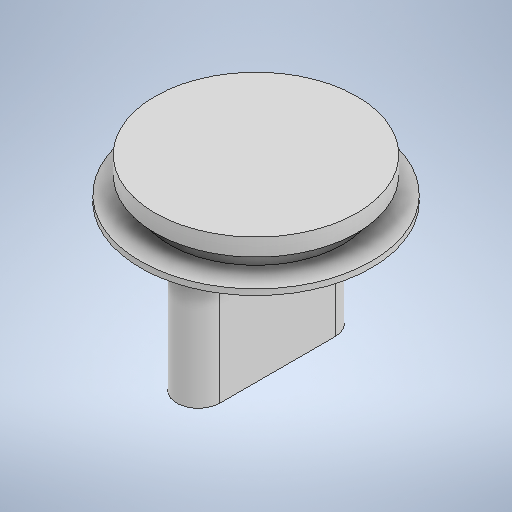
# Autodesk Inventor part: Pin Hole Lock
Saved by Autodesk Inventor 2025 (Build 290162010, 162A)
## iProperties
Created: 2024-06-11
Part Number: Pin Hole Lock
Material: Generic
Document SubType Name: Modeling
Designer: vncnt
Density: 1 g/cm^3
Appearance: Default
Author: vncnt
Autodesk Inventor part; units mm, degrees
ref_plane "YZ Plane" through (0, 0, 0) normal (1, 0, 0) x (0, 1, 0)
ref_plane "XZ Plane" through (0, 0, 0) normal (0, 1, 0) x (-1, 0, 0)
ref_plane "XY Plane" through (0, 0, 0) normal (0, 0, 1) x (1, 0, 0)
sketch "Sketch1" plane through (0, 0, 0) normal (0, 1, 0) x (-1, 0, 0)
  circle A0 centre (0, 0) radius 1.905
  dimension "d0" = 3.81
  constraints: 1 centre point, 1 coincident
  measures "d0" diameter of A0
extrude "Extrusion1" add sketch "Sketch1" along normal blind 2.341
sketch "Sketch2" plane through (0, 2.341, 0) normal (0, 1, 0) x (1, 0, 0)
  circle A0 centre (0, 0) radius 2
  dimension "d3" = 4
  constraints: 1 centre point, 1 coincident
  measures "d3" diameter of A0
extrude "Extrusion2" add sketch "Sketch2" along normal blind 0.1
sketch "Sketch8" plane through (0, 0, 0) normal (0, -1, 0) x (1, 0, 0)
  line L0 (0, 1) -> (0, -1) construction
  line L1 (-0.375, 1) -> (-0.375, -1)
  line L2 (0.375, -1) -> (0.375, 1)
  arc A0 (0.375, 1) -> (-0.375, 1) centre (0, 1) ccw
  arc A1 (-0.375, -1) -> (0.375, -1) centre (0, -1) ccw
  circle A2 centre (0, 0) radius 1.905
  dimension "d22" = 1
  dimension "d23" = 0.75
  constraints: 8 end point, 4 point on circle, 4 tangent, 3 centre point, 1 coincident, 1 midpoint, 1 parallel, 1 vertical
  measures "d22" distance of point (0, 0) L0.end
  measures "d23" diameter of A1
extrude "Extrusion4" cut sketch "Sketch8" against normal up to surface (2.341 mm away)
sketch "Sketch9" plane through (0, 2.441, 0) normal (0, 1, 0) x (1, 0, 0)
  circle A0 centre (0, 0) radius 1.5
  dimension "d26" = 3
  constraints: 1 centre point, 1 coincident
  measures "d26" diameter of A0
extrude "Extrusion5" add sketch "Sketch9" along normal blind 0.3
sketch "Sketch10" plane through (0, 2.741, 0) normal (0, 1, 0) x (1, 0, 0)
  circle A0 centre (0, 0) radius 1.75
  dimension "d29" = 3.5
  constraints: 1 centre point, 1 coincident
  measures "d29" diameter of A0
extrude "Extrusion6" add sketch "Sketch10" along normal blind 0.3
body "Solid1"
